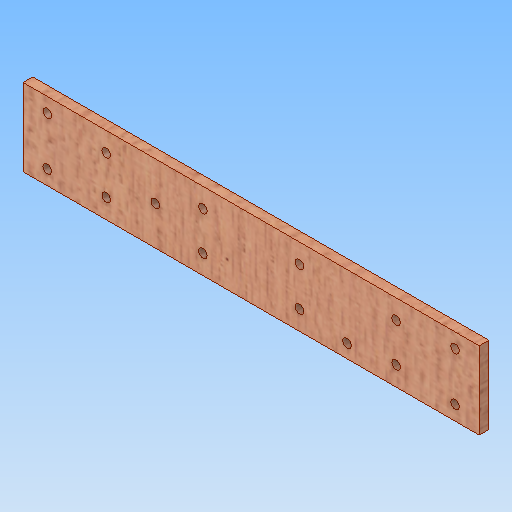
# Autodesk Inventor part: Top_Slider Piece 1_4 Lanes
Saved by Autodesk Inventor 2018.1 (Build 221171000, 171)
## iProperties
Created: 2019-03-18
Part Number: Top_Slider Piece 1_4 Lanes
Material: Wood (Oak)
Document SubType Name: Modeling
Designer: James
Density: 0.76 g/cm^3
Appearance: White Oak - Natural Medium Gloss
Mass: 35.0259 g
Surface Area: 221.843 cm^2
Volume: 46.0867 cm^3
Author: James
Autodesk Inventor part; units mm, degrees
ref_plane "YZ Plane" through (0, 0, 0) normal (1, 0, 0) x (0, 1, 0)
ref_plane "XZ Plane" through (0, 0, 0) normal (0, 1, 0) x (-1, 0, 0)
ref_plane "XY Plane" through (0, 0, 0) normal (0, 0, 1) x (1, 0, 0)
sketch "Sketch1" plane through (0, 0, 0) normal (0, 0, 1) x (1, 0, 0)
  line L0 (0, 0) -> (236, 0)
  line L1 (236, 0) -> (236, 40)
  line L2 (236, 40) -> (0, 40)
  line L3 (0, 40) -> (0, 0)
  dimension "d0" = 236
  dimension "d1" = 40
  constraints: 8 end point, 2 parallel, 1 horizontal, 1 perpendicular
  measures "d0" distance of L2.end L1.end
  measures "d1" distance of L1.end L0.end
extrude "Extrusion1" add sketch "Sketch1" along normal blind 5
sketch "Sketch2" plane through (0, 0, 5) normal (0, 0, 1) x (1, 0, 0)
  line L0 (236, 40) -> (0, 40) projected
  line L1 (0, 0) -> (236, 0) projected
  line L2 (0, 40) -> (0, 0) projected
  point P0 (43, 30)
  point P1 (43, 10)
  dimension "d4" = 10
  dimension "d6" = 43
  dimension "d40" = 20
  dimension "d41" = 10
  constraints: 1 vertical alignment
  measures "d4" distance from line of L0 point (43, 30)
  measures "d6" distance from line of point (43, 30) L2
  measures "d40" distance of point (43, 10) point (43, 30)
  measures "d41" distance from line of L1 point (43, 10)
hole "Hole1" at (43, 30, 5) at (43, 10, 5) direction (0, 0, -1) diameter 4.5 end through all clearance for "Flat Head Machine Screw" size "M4" standard "Ansi Metric M Profile"
pattern_linear "Rectangular Pattern1" count 4 spacing 50 along (1, 0, 0) of "Hole1"
sketch "Sketch3" plane through (0, 0, 5) normal (0, 0, 1) x (1, 0, 0)
  line L0 (236, 40) -> (0, 40) projected
  line L1 (0, 40) -> (0, 0) projected
  line L2 (236, 0) -> (236, 40) projected
  point P0 (68.4243, 20)
  point P1 (167.5757, 7)
  dimension "d17" = 100
  dimension "d18" = 20
  dimension "d19" = 13
  dimension "d20" = 68.4243
  dimension "d21" = 68.4243
  measures "d17" distance of point (167.576, 7) point (68.424, 20)
  measures "d18" distance from line of L0 point (68.424, 20)
  measures "d19" vertical distance of point (68.424, 20) point (167.576, 7)
  measures "d20" distance from line of L1 point (68.424, 20)
  measures "d21" distance from line of L2 point (167.576, 7)
hole "Hole2" at (68.4243, 20, 5) at (167.5757, 7, 5) direction (0, 0, -1) diameter 4.5 end through all clearance for "Flat Head Machine Screw" size "M4" standard "Ansi Metric M Profile"
sketch "Sketch4" plane through (0, 0, 5) normal (0, 0, 1) x (1, 0, 0)
  line L0 (236, 40) -> (0, 40) projected
  line L1 (0, 0) -> (236, 0) projected
  line L2 (0, 40) -> (0, 0) projected
  line L3 (236, 0) -> (236, 40) projected
  point P0 (12.5, 32.5)
  point P1 (12.5, 7.5)
  point P2 (223.5, 32.5)
  point P3 (223.5, 7.5)
  dimension "d29" = 7.5
  dimension "d30" = 7.5
  dimension "d31" = 12.5
  dimension "d32" = 12.5
  constraints: 2 horizontal alignment, 2 vertical alignment
  measures "d29" distance from line of L0 point (12.5, 32.5)
  measures "d30" distance from line of L1 point (12.5, 7.5)
  measures "d31" distance from line of L2 point (12.5, 32.5)
  measures "d32" distance from line of L3 point (223.5, 32.5)
hole "Hole3" at (12.5, 32.5, 5) at (12.5, 7.5, 5) at (223.5, 32.5, 5) at (223.5, 7.5, 5) direction (0, 0, -1) diameter 4.5 end through all clearance for "Flat Head Machine Screw" size "M4" standard "Ansi Metric M Profile"
equation "\"d20\" = d21"
equation "\"d30\" = d29"
equation "\"d32\" = d31"
body "Solid1"
